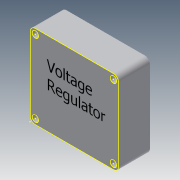
# Autodesk Inventor part: voltage Regulator
Saved by Autodesk Inventor 2014 (Build 180170000, 170)
## iProperties
Created: 2016-01-12
Part Number: voltage Regulator
Material: Generic
Document SubType Name: Modeling
Designer: Paul
Density: 1 g/cm^3
Appearance: Default
Author: Paul
Autodesk Inventor part; units mm, degrees
ref_plane "YZ Plane" through (0, 0, 0) normal (1, 0, 0) x (0, 1, 0)
ref_plane "XZ Plane" through (0, 0, 0) normal (0, 1, 0) x (-1, 0, 0)
ref_plane "XY Plane" through (0, 0, 0) normal (0, 0, 1) x (1, 0, 0)
sketch "Sketch1" plane through (0, 0, 0) normal (0, 0, 1) x (1, 0, 0)
  line L0 (3.175, 0) -> (50.8, 0)
  line L1 (53.975, 3.175) -> (53.975, 47.625)
  line L2 (50.8, 50.8) -> (3.175, 50.8)
  line L3 (0, 47.625) -> (0, 3.175)
  arc A0 (0, 3.175) -> (3.175, 0) centre (3.175, 3.175) ccw
  arc A1 (3.175, 50.8) -> (0, 47.625) centre (3.175, 47.625) ccw
  arc A2 (53.975, 47.625) -> (50.8, 50.8) centre (50.8, 47.625) ccw
  arc A3 (50.8, 0) -> (53.975, 3.175) centre (50.8, 3.175) ccw
  circle A4 centre (3.175, 47.625) radius 1.9812
  circle A5 centre (3.175, 3.175) radius 1.9812
  circle A6 centre (50.8, 3.175) radius 1.9812
  circle A7 centre (50.8, 47.625) radius 1.9812
  point P0 (0, 0)
  point P1 (53.975, 50.8)
  point P2 (53.975, 0)
  point P3 (0, 50.8)
  dimension "d0" = 53.975
  dimension "d1" = 50.8
  dimension "d2" = 3.175
  dimension "d3" = 3.9624
  constraints: 8 centre point, 8 end point, 8 point on circle, 8 point on line, 8 tangent, 6 equal radius, 4 coincident, 2 parallel, 1 horizontal, 1 perpendicular
  measures "d0" distance of point (0, 50.8) point (53.975, 50.8)
  measures "d1" distance of point (53.975, 50.8) point (53.975, 0)
  measures "d2" radius of A0
  measures "d3" diameter of A4
extrude "Extrusion1" add sketch "Sketch1" along normal blind 19.05
sketch "Sketch2" plane through (0, 0, 19.05) normal (0, 0, 1) x (1, 0, 0)
  circle A0 centre (50.8, 47.625) radius 1.9812 projected
  circle A1 centre (50.8, 3.175) radius 1.9812 projected
  circle A2 centre (3.175, 3.175) radius 1.9812 projected
  circle A3 centre (3.175, 47.625) radius 1.9812 projected
  line L0 (3.175, 0) -> (50.8, 0) projected
  arc A4 (50.8, 0) -> (53.975, 3.175) centre (50.8, 3.175) ccw projected
  line L1 (53.975, 3.175) -> (53.975, 47.625) projected
  arc A5 (53.975, 47.625) -> (50.8, 50.8) centre (50.8, 47.625) ccw projected
  line L2 (50.8, 50.8) -> (3.175, 50.8) projected
  arc A6 (3.175, 50.8) -> (0, 47.625) centre (3.175, 47.625) ccw projected
  line L3 (0, 47.625) -> (0, 3.175) projected
  arc A7 (0, 3.175) -> (3.175, 0) centre (3.175, 3.175) ccw projected
  line L4 (10.2285, 38.5195) -> (40.5302, 38.5195) construction
  line L5 (40.5302, 38.5195) -> (40.5302, 16.6819) construction
  line L6 (40.5302, 16.6819) -> (10.2285, 16.6819) construction
  line L7 (10.2285, 16.6819) -> (10.2285, 38.5195) construction
  point P0 (0, 0)
  constraints: 2 other
body "Solid1"
